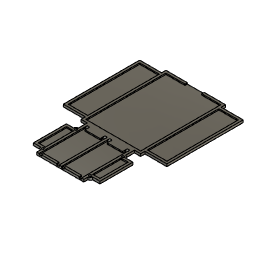
RodogCompartmentsV1 (Autodesk Fusion 360 design; units mm, degrees)
Autodesk Fusion 360 part; units mm, degrees
note: some values were not read from the file. Chosen so that the rebuilt part matches the saved one: which pieces of a blend or face edit are solid. Set by a fixed rule: which sketch regions a step uses.
sketch "Sketch1" plane through (0, 0, 0) normal (0, 0, 1) x (1, 0, 0)
sketch "Sketch2" plane through (0, 0, 0) normal (0, 0, 1) x (1, 0, 0)
  line L0 (25.146, 24.384) -> (-25.146, 24.384)
  line L1 (-25.146, 24.384) -> (-25.146, -24.384)
  line L2 (-25.146, -24.384) -> (25.146, -24.384)
  line L3 (25.146, -24.384) -> (25.146, 24.384)
  line L4 (25.146, 24.384) -> (-25.146, -24.384) construction
  line L5 (-25.146, 24.384) -> (25.146, -24.384) construction
  dimension "d3" = 50.292
  dimension "d4" = 48.768
  constraint horizontal L0
  constraint perpendicular L0 L1
  constraint parallel L0 L2
  constraint parallel L1 L3
  constraint coincident L4 origin
  constraint coincident L5 origin
  measures "d3" distance of L1.end L2.end
  measures "d4" distance of L0.end L1.end
extrude "Extrude1" add sketch "Sketch2" along normal blind 2.54 makes body 1
sketch "Sketch3" plane through (0, 0, 2.54) normal (0, 0, 1) x (-1, 0, 0)
  line L0 (-25.146, 24.384) -> (-25.146, -24.384)
  line L1 (-25.146, -24.384) -> (25.146, -24.384)
  line L2 (25.146, -24.384) -> (25.146, 24.384)
  line L3 (25.146, 24.384) -> (-25.146, 24.384)
  line L4 (-25.146, 24.384) -> (-22.606, 24.384)
  line L5 (-22.606, 24.384) -> (-22.606, 21.844)
  line L6 (-22.606, 21.844) -> (-25.146, 21.844)
  line L7 (-25.146, 21.844) -> (-25.146, 24.384)
  line L8 (-22.606, 21.844) -> (-1.27, 21.844)
  line L9 (-1.27, 21.844) -> (-1.27, -21.844)
  line L10 (-1.27, -21.844) -> (-22.606, -21.844)
  line L11 (-22.606, -21.844) -> (-22.606, 21.844)
  line L12 (-1.27, 21.844) -> (1.27, 21.844)
  line L13 (1.27, 21.844) -> (22.606, 21.844)
  line L14 (22.606, 21.844) -> (22.606, -21.844)
  line L15 (22.606, -21.844) -> (1.27, -21.844)
  line L16 (1.27, -21.844) -> (1.27, 21.844)
  dimension "d7" = 2.54
  dimension "d8" = 2.54
  dimension "d9" = 21.336
  dimension "d10" = 43.688
  dimension "d11" = 2.54
  dimension "d12" = 21.336
  dimension "d13" = 43.688
  constraint horizontal L4
  constraint vertical L5
  constraint horizontal L6
  constraint vertical L7
  constraint coincident L0.start L3.end
  constraint horizontal L8
  constraint vertical L9
  constraint horizontal L10
  constraint vertical L11
  constraint perpendicular L9 L12
  constraint horizontal L13
  constraint vertical L14
  constraint horizontal L15
  constraint vertical L16
  measures "d7" distance of L0.start L4.end
  measures "d8" distance of L0.start L6.end
  measures "d9" distance of L5.end L8.end
  measures "d10" distance of L5.end L10.end
  measures "d11" distance of L8.end L12.end
  measures "d12" distance of L12.end L13.end
  measures "d13" distance of L12.end L15.end
extrude "Extrude2" cut sketch "Sketch3" against normal blind 1.27 contours L8 L9 L10 L11 | L13 L14 L15 L16 bodies 1
sketch "Sketch4" plane through (0, 0, 2.54) normal (0, 0, 1) x (-1, 0, 0)
  line L0 (-1.27, 21.844) -> (-1.27, -21.844)
  line L1 (-1.27, -21.844) -> (-22.606, -21.844)
  line L2 (-22.606, -21.844) -> (-22.606, 21.844)
  line L3 (-22.606, 21.844) -> (-1.27, 21.844)
  line L4 (22.606, 21.844) -> (22.606, -21.844)
  line L5 (22.606, -21.844) -> (1.27, -21.844)
  line L6 (1.27, -21.844) -> (1.27, 21.844)
  line L7 (1.27, 21.844) -> (22.606, 21.844)
  line L8 (-25.146, 24.384) -> (-25.146, -24.384)
  line L9 (-25.146, -24.384) -> (25.146, -24.384)
  line L10 (25.146, -24.384) -> (25.146, 24.384)
  line L11 (25.146, 24.384) -> (-25.146, 24.384)
  line L12 (-22.606, 21.844) -> (-20.066, 21.844)
  line L13 (-20.066, 21.844) -> (-20.066, 24.384)
  line L14 (-20.066, 24.384) -> (-22.606, 24.384)
  line L15 (-22.606, 24.384) -> (-22.606, 21.844)
  line L16 (-1.27, 21.844) -> (-3.81, 21.844)
  line L17 (-3.81, 21.844) -> (-3.81, 24.384)
  line L18 (-3.81, 24.384) -> (-1.27, 24.384)
  line L19 (-1.27, 24.384) -> (-1.27, 21.844)
  line L20 (-22.606, -21.844) -> (-20.066, -21.844)
  line L21 (-20.066, -21.844) -> (-20.066, -24.384)
  line L22 (-20.066, -24.384) -> (-22.606, -24.384)
  line L23 (-22.606, -24.384) -> (-22.606, -21.844)
  line L24 (-1.27, -21.844) -> (-3.81, -21.844)
  line L25 (-3.81, -21.844) -> (-3.81, -24.384)
  line L26 (-3.81, -24.384) -> (-1.27, -24.384)
  line L27 (-1.27, -24.384) -> (-1.27, -21.844)
  dimension "d16" = 2.54
  dimension "d17" = 2.54
  dimension "d18" = 2.54
  dimension "d19" = 2.54
  dimension "d20" = 2.54
  dimension "d21" = 2.54
  constraint horizontal L12
  constraint vertical L13
  constraint horizontal L14
  constraint vertical L15
  constraint coincident L2.end L3.start
  constraint horizontal L16
  constraint vertical L17
  constraint horizontal L18
  constraint vertical L19
  constraint coincident L0.start L3.end
  constraint horizontal L20
  constraint vertical L21
  constraint horizontal L22
  constraint vertical L23
  constraint coincident L1.end L2.start
  constraint horizontal L24
  constraint vertical L25
  constraint horizontal L26
  constraint vertical L27
  constraint coincident L0.end L1.start
  measures "d16" distance of L2.end L12.end
  measures "d17" distance of L0.start L16.end
  measures "d18" distance of L0.start L18.end
  measures "d19" distance of L1.end L20.end
  measures "d20" distance of L1.end L22.end
  measures "d21" distance of L0.end L24.end
extrude "Extrude3" cut sketch "Sketch4" against normal blind 1.27 contours L3 L11 L16 L17 L18 L19 | L1 L9 L24 L25 L26 L27 | L3 L11 L12 L13 L14 L15 | L1 L9 L20 L21 L22 L23 bodies 1
sketch "Sketch5" plane through (0, 0, 2.54) normal (0, 0, 1) x (-1, 0, 0)
  line L0 (-1.27, 24.384) -> (-1.27, -24.384)
  line L1 (-1.27, -24.384) -> (25.146, -24.384)
  line L2 (25.146, -24.384) -> (25.146, 24.384)
  line L3 (25.146, 24.384) -> (-1.27, 24.384)
  line L4 (22.606, 21.844) -> (22.606, -21.844)
  line L5 (22.606, -21.844) -> (1.27, -21.844)
  line L6 (1.27, -21.844) -> (1.27, 21.844)
  line L7 (1.27, 21.844) -> (22.606, 21.844)
  line L8 (1.27, 21.844) -> (3.81, 21.844)
  line L9 (3.81, 21.844) -> (3.81, 24.384)
  line L10 (3.81, 24.384) -> (1.27, 24.384)
  line L11 (1.27, 24.384) -> (1.27, 21.844)
  line L12 (22.606, 21.844) -> (20.066, 21.844)
  line L13 (20.066, 21.844) -> (20.066, 24.384)
  line L14 (20.066, 24.384) -> (22.606, 24.384)
  line L15 (22.606, 24.384) -> (22.606, 21.844)
  line L16 (1.27, -21.844) -> (3.81, -21.844)
  line L17 (3.81, -21.844) -> (3.81, -24.384)
  line L18 (3.81, -24.384) -> (1.27, -24.384)
  line L19 (1.27, -24.384) -> (1.27, -21.844)
  line L20 (22.606, -21.844) -> (20.066, -21.844)
  line L21 (20.066, -21.844) -> (20.066, -24.384)
  line L22 (20.066, -24.384) -> (22.606, -24.384)
  line L23 (22.606, -24.384) -> (22.606, -21.844)
  dimension "d24" = 2.54
  dimension "d25" = 2.54
  dimension "d26" = 2.54
  dimension "d27" = 2.54
  constraint horizontal L8
  constraint vertical L9
  constraint horizontal L10
  constraint vertical L11
  constraint coincident L6.end L7.start
  constraint horizontal L12
  constraint vertical L13
  constraint horizontal L14
  constraint vertical L15
  constraint coincident L4.start L7.end
  constraint horizontal L16
  constraint vertical L17
  constraint horizontal L18
  constraint vertical L19
  constraint coincident L5.end L6.start
  constraint horizontal L20
  constraint vertical L21
  constraint horizontal L22
  constraint vertical L23
  constraint coincident L4.end L5.start
  measures "d24" distance of L6.end L8.end
  measures "d25" distance of L4.start L12.end
  measures "d26" distance of L5.end L16.end
  measures "d27" distance of L4.end L20.end
extrude "Extrude4" cut sketch "Sketch5" against normal blind 1.27 contours L3 L7 L8 L9 L10 L11 | L1 L5 L16 L17 L18 L19 | L3 L7 L12 L13 L14 L15 | L1 L5 L20 L21 L22 L23 bodies 1
sketch "Sketch6" plane through (25.146, 0, 0) normal (1, 0, 0) x (0, 1, 0)
  line L0 (-24.384, 0) -> (24.384, 0)
  line L1 (24.384, 0) -> (24.384, 2.54)
  line L2 (24.384, 2.54) -> (-24.384, 2.54)
  line L3 (-24.384, 2.54) -> (-24.384, 0)
  line L4 (-24.384, 2.54) -> (0, 2.54)
  line L5 (0, 2.54) -> (0, 1.27)
  line L6 (15.0368, 2.54) -> (-15.0368, 2.54)
  line L7 (-15.0368, 2.54) -> (-15.0368, 0)
  line L8 (-15.0368, 0) -> (15.0368, 0)
  line L9 (15.0368, 0) -> (15.0368, 2.54)
  line L10 (15.0368, 2.54) -> (-15.0368, 0) construction
  line L11 (-15.0368, 2.54) -> (15.0368, 0) construction
  point P0 (0, 1.27)
  dimension "d30" = 24.384
  dimension "d31" = 1.27
  dimension "d32" = 30.0736
  dimension "d33" = 2.54
  constraint coincident L2.end L3.start
  constraint perpendicular L3 L4
  constraint perpendicular L4 L5
  constraint horizontal L6
  constraint perpendicular L6 L7
  constraint parallel L6 L8
  constraint parallel L7 L9
  constraint coincident L10 P0
  constraint coincident L11 P0
  constraint coincident P0 L5.end
  measures "d30" distance of L2.end L4.end
  measures "d31" distance of L4.end P0
  measures "d32" distance of L7.end L8.end
  measures "d33" distance of L6.end L7.end
extrude "Extrude5" add sketch "Sketch6" along normal blind 10.287 contours L0 L2 L4 L6 L7 L8 L9 bodies 1
extrude "Extrude6" add 1 faces at (28.575, -15.0368, 1.6933) along direction (0, -1, 0) blind 2.54 on bodies 1 bodies 1
extrude "Extrude7" add 1 faces at (28.575, 15.0368, 0.8467) along direction (0, 1, 0) blind 2.54 on bodies 1 bodies 1
sketch "Sketch7" plane through (0, 0, 2.54) normal (0, 0, 1) x (-1, 0, 0)
  line L0 (-22.606, -24.384) -> (-22.606, 24.384)
  line L1 (-22.606, 24.384) -> (-25.146, 24.384)
  line L2 (-25.146, 24.384) -> (-25.146, 17.5768)
  line L3 (-25.146, 17.5768) -> (-35.433, 17.5768)
  line L4 (-35.433, 17.5768) -> (-35.433, -17.5768)
  line L5 (-35.433, -17.5768) -> (-25.146, -17.5768)
  line L6 (-25.146, -17.5768) -> (-25.146, -24.384)
  line L7 (-25.146, -24.384) -> (-22.606, -24.384)
  line L8 (-35.433, 17.5768) -> (-32.893, 17.5768)
  line L9 (-32.893, 17.5768) -> (-32.893, 15.0368)
  line L10 (-32.893, 15.0368) -> (-35.433, 15.0368)
  line L11 (-35.433, 15.0368) -> (-35.433, 17.5768)
  line L12 (-32.893, 15.0368) -> (-25.146, 15.0368)
  line L13 (-25.146, 15.0368) -> (-25.146, -15.0368)
  line L14 (-25.146, -15.0368) -> (-32.893, -15.0368)
  line L15 (-32.893, -15.0368) -> (-32.893, 15.0368)
  dimension "d40" = 2.54
  dimension "d41" = 2.54
  dimension "d42" = 7.747
  dimension "d43" = 30.0736
  constraint horizontal L8
  constraint vertical L9
  constraint horizontal L10
  constraint vertical L11
  constraint coincident L3.end L4.start
  constraint horizontal L12
  constraint vertical L13
  constraint horizontal L14
  constraint vertical L15
  measures "d40" distance of L3.end L8.end
  measures "d41" distance of L3.end L10.end
  measures "d42" distance of L9.end L12.end
  measures "d43" distance of L9.end L14.end
extrude "Extrude8" cut sketch "Sketch7" against normal blind 1.27 contours L12 L13 L14 L15 bodies 1
sketch "Sketch8" plane through (-25.146, 0, 0) normal (-1, 0, 0) x (0, -1, 0)
  line L0 (-24.384, 0) -> (24.384, 0)
  line L1 (24.384, 0) -> (24.384, 2.54)
  line L2 (24.384, 2.54) -> (-24.384, 2.54)
  line L3 (-24.384, 2.54) -> (-24.384, 0)
  line L4 (-24.384, 2.54) -> (0, 2.54)
  line L5 (0, 2.54) -> (0, 1.27)
  line L6 (-17.5768, 0) -> (17.5768, 0)
  line L7 (17.5768, 0) -> (17.5768, 2.54)
  line L8 (17.5768, 2.54) -> (-17.5768, 2.54)
  line L9 (-17.5768, 2.54) -> (-17.5768, 0)
  line L10 (-17.5768, 0) -> (17.5768, 2.54) construction
  line L11 (17.5768, 0) -> (-17.5768, 2.54) construction
  point P0 (0, 1.27)
  dimension "d46" = 24.384
  dimension "d47" = 1.27
  dimension "d48" = 35.1536
  constraint coincident L2.end L3.start
  constraint perpendicular L3 L4
  constraint perpendicular L4 L5
  constraint horizontal L6
  constraint perpendicular L6 L7
  constraint parallel L6 L8
  constraint parallel L7 L9
  constraint coincident L10 P0
  constraint coincident L11 P0
  constraint coincident P0 L5.end
  measures "d46" distance of L2.end L4.end
  measures "d47" distance of L4.end P0
  measures "d48" distance of L7.end L8.end
extrude "Extrude9" add sketch "Sketch8" along normal blind 10.287 contours L0 L2 L4 L6 L7 L8 L9 bodies 1
sketch "Sketch9" plane through (0, 0, 2.54) normal (0, 0, 1) x (-1, 0, 0)
  line L0 (22.606, 24.384) -> (22.606, -24.384)
  line L1 (22.606, -24.384) -> (25.146, -24.384)
  line L2 (25.146, -24.384) -> (25.146, -17.5768)
  line L3 (25.146, -17.5768) -> (35.433, -17.5768)
  line L4 (35.433, -17.5768) -> (35.433, 17.5768)
  line L5 (35.433, 17.5768) -> (25.146, 17.5768)
  line L6 (25.146, 17.5768) -> (25.146, 24.384)
  line L7 (25.146, 24.384) -> (22.606, 24.384)
  line L8 (35.433, 17.5768) -> (32.893, 17.5768)
  line L9 (32.893, 17.5768) -> (32.893, 15.0368)
  line L10 (32.893, 15.0368) -> (35.433, 15.0368)
  line L11 (35.433, 15.0368) -> (35.433, 17.5768)
  line L12 (32.893, 15.0368) -> (24.003, 15.0368)
  line L13 (24.003, 15.0368) -> (24.003, -15.0368)
  line L14 (24.003, -15.0368) -> (32.893, -15.0368)
  line L15 (32.893, -15.0368) -> (32.893, 15.0368)
  dimension "d51" = 2.54
  dimension "d52" = 2.54
  dimension "d53" = 8.89
  dimension "d54" = 30.0736
  constraint horizontal L8
  constraint vertical L9
  constraint horizontal L10
  constraint vertical L11
  constraint coincident L4.end L5.start
  constraint horizontal L12
  constraint vertical L13
  constraint horizontal L14
  constraint vertical L15
  measures "d51" distance of L4.end L8.end
  measures "d52" distance of L4.end L10.end
  measures "d53" distance of L9.end L12.end
  measures "d54" distance of L9.end L14.end
extrude "Extrude10" cut sketch "Sketch9" against normal blind 1.27 contours L12 L13 L14 L15 bodies 1
extrude "Extrude11" add 1 faces at (-26.9663, -5.0123, 1.27) along direction (0, 0, 1) blind 1.27 on bodies 1 bodies 1
sketch "Sketch11" plane through (0, 0, 2.54) normal (0, 0, 1) x (-1, 0, 0)
  line L0 (22.606, 24.384) -> (22.606, -24.384)
  line L1 (22.606, -24.384) -> (25.146, -24.384)
  line L2 (25.146, -24.384) -> (25.146, -17.5768)
  line L3 (25.146, -17.5768) -> (35.433, -17.5768)
  line L4 (35.433, -17.5768) -> (35.433, 17.5768)
  line L5 (35.433, 17.5768) -> (25.146, 17.5768)
  line L6 (25.146, 17.5768) -> (25.146, 24.384)
  line L7 (25.146, 24.384) -> (22.606, 24.384)
  line L8 (35.433, -17.5768) -> (32.893, -17.5768)
  line L9 (32.893, -17.5768) -> (32.893, -15.0368)
  line L10 (32.893, -15.0368) -> (35.433, -15.0368)
  line L11 (35.433, -15.0368) -> (35.433, -17.5768)
  line L12 (32.893, -15.0368) -> (25.146, -15.0368)
  line L13 (25.146, -15.0368) -> (25.146, 15.0368)
  line L14 (25.146, 15.0368) -> (32.893, 15.0368)
  line L15 (32.893, 15.0368) -> (32.893, -15.0368)
  dimension "d59" = 2.54
  dimension "d60" = 2.54
  dimension "d61" = 7.747
  dimension "d62" = 30.0736
  constraint horizontal L8
  constraint vertical L9
  constraint horizontal L10
  constraint vertical L11
  constraint coincident L3.end L4.start
  constraint horizontal L12
  constraint vertical L13
  constraint horizontal L14
  constraint vertical L15
  measures "d59" distance of L3.end L8.end
  measures "d60" distance of L3.end L10.end
  measures "d61" distance of L9.end L12.end
  measures "d62" distance of L9.end L14.end
extrude "Extrude12" cut sketch "Sketch11" against normal blind 1.27 contours L12 L13 L14 L15 bodies 1
sketch "Sketch13" plane through (0, 17.5768, 0) normal (0, 1, 0) x (-1, 0, 0)
  line L0 (25.146, 2.54) -> (25.146, 0)
  line L1 (25.146, 0) -> (35.433, 0)
  line L2 (35.433, 0) -> (35.433, 2.54)
  line L3 (35.433, 2.54) -> (25.146, 2.54)
  line L4 (25.146, 2.54) -> (27.686, 2.54)
  line L5 (27.686, 2.54) -> (27.686, 0)
  line L6 (27.686, 0) -> (25.146, 0)
  line L7 (25.146, 0) -> (25.146, 2.54)
  dimension "d65" = 2.54
  constraint horizontal L4
  constraint vertical L5
  constraint horizontal L6
  constraint vertical L7
  constraint coincident L0.start L3.end
  measures "d65" distance of L0.start L4.end
extrude "Extrude13" add sketch "Sketch13" along normal blind 2.54 contours L0 L1 L3 L4 L5 L6 L7 bodies 1
sketch "Sketch14" plane through (0, 0, 2.54) normal (0, 0, 1) x (-1, 0, 0)
  circle A0 centre (25.146, -17.5768) radius 1.27
  point P0 (25.146, -17.5768)
  dimension "d68" = 2.54
  constraint coincident P0 A0.centre
  measures "d68" diameter of A0
extrude "Extrude14" cut sketch "Sketch14" against normal blind 1.27 bodies 1
fillet "Fillet1" radius 2.54 1 edges at (-27.686, 20.1168, 1.27) on bodies 1
sketch "Sketch15" plane through (25.146, 0, 0) normal (1, 0, 0) x (0, 1, 0)
  line L0 (17.5768, 2.54) -> (17.5768, 0)
  line L1 (17.5768, 0) -> (24.384, 0)
  line L2 (24.384, 0) -> (24.384, 2.54)
  line L3 (24.384, 2.54) -> (17.5768, 2.54)
  line L4 (17.5768, 2.54) -> (20.1168, 2.54)
  line L5 (20.1168, 2.54) -> (20.1168, 0)
  line L6 (20.1168, 0) -> (17.5768, 0)
  line L7 (17.5768, 0) -> (17.5768, 2.54)
  dimension "d73" = 2.54
  constraint horizontal L4
  constraint vertical L5
  constraint horizontal L6
  constraint vertical L7
  constraint coincident L0.start L3.end
  measures "d73" distance of L0.start L4.end
extrude "Extrude15" add sketch "Sketch15" along normal blind 2.54 contours L0 L1 L3 L4 L5 L6 L7 bodies 1
sketch "Sketch16" plane through (25.146, 0, 0) normal (1, 0, 0) x (0, 1, 0)
  line L0 (-17.5768, 0) -> (-17.5768, 2.54)
  line L1 (-17.5768, 2.54) -> (-24.384, 2.54)
  line L2 (-24.384, 2.54) -> (-24.384, 0)
  line L3 (-24.384, 0) -> (-17.5768, 0)
  line L4 (-17.5768, 2.54) -> (-20.1168, 2.54)
  line L5 (-20.1168, 2.54) -> (-20.1168, 0)
  line L6 (-20.1168, 0) -> (-17.5768, 0)
  line L7 (-17.5768, 0) -> (-17.5768, 2.54)
  dimension "d76" = 2.54
  constraint horizontal L4
  constraint vertical L5
  constraint horizontal L6
  constraint vertical L7
  constraint coincident L0.end L1.start
  measures "d76" distance of L0.end L4.end
extrude "Extrude16" add sketch "Sketch16" along normal blind 2.54 contours L0 L1 L3 L4 L5 L6 L7 bodies 1
sketch "Sketch17" plane through (-25.146, 0, 0) normal (-1, 0, 0) x (0, -1, 0)
  line L0 (17.5768, 2.54) -> (17.5768, 0)
  line L1 (17.5768, 0) -> (24.384, 0)
  line L2 (24.384, 0) -> (24.384, 2.54)
  line L3 (24.384, 2.54) -> (17.5768, 2.54)
  line L4 (17.5768, 2.54) -> (20.1168, 2.54)
  line L5 (20.1168, 2.54) -> (20.1168, 0)
  line L6 (20.1168, 0) -> (17.5768, 0)
  line L7 (17.5768, 0) -> (17.5768, 2.54)
  dimension "d79" = 2.54
  constraint horizontal L4
  constraint vertical L5
  constraint horizontal L6
  constraint vertical L7
  constraint coincident L0.start L3.end
  measures "d79" distance of L0.start L4.end
extrude "Extrude17" add sketch "Sketch17" along normal blind 2.54 contours L0 L1 L3 L4 L5 L6 L7 bodies 1
sketch "Sketch18" plane through (0, 0, 2.54) normal (0, 0, 1) x (-1, 0, 0)
  line L0 (35.433, 17.5768) -> (25.146, 17.5768)
  line L1 (22.606, 24.384) -> (22.606, -24.384)
  line L2 (27.7188, 17.5768) -> (22.606, 17.5768)
  circle A0 centre (25.146, 17.5768) radius 1.27
  line L3 (-27.686, 17.526) -> (-22.606, 17.526)
  circle A1 centre (-25.146, 17.526) radius 1.27
  line L4 (-27.686, -17.526) -> (-22.606, -17.526)
  circle A2 centre (-25.146, -17.526) radius 1.27
  dimension "d82" = 2.54
  dimension "d83" = 2.54
  dimension "d84" = 2.54
  constraint coincident L0 L2.start
  constraint coincident L1 L2.end
  constraint perpendicular L1 L2
  constraint coincident L0.end A0.centre
  constraint horizontal L3
  constraint midpoint L3 A1.centre
  constraint horizontal L4
  constraint midpoint L4 A2.centre
  measures "d82" diameter of A0
  measures "d83" diameter of A1
  measures "d84" diameter of A2
extrude "Extrude18" cut sketch "Sketch18" against normal blind 1.27 bodies 1
fillet "Fillet2" radius 2.54 3 edges at (-27.686, -20.1168, 1.27) (27.686, -20.1168, 1.27) (27.686, 20.1168, 1.27) on bodies 1
sketch "Sketch20" plane through (0, 0, 0) normal (0, 0, 1) x (1, 0, 0)
  circle A0 centre (63.5, 12.7) radius 1.27
  dimension "d89" = 2.54
  measures "d89" diameter of A0
extrude "Extrude19" add sketch "Sketch20" along normal blind 18.034 separate body makes body 2
move_face "MoveFace1" to x (1, 0, 0) y (0, 1, 0) z (0, 0, 1) at (-25.4, 0, 0) 1 faces at (64.0223, 13.8576, 12.0227) on bodies 2
sketch "Sketch23" plane through (0, 0, 0) normal (0, 0, 1) x (1, 0, 0)
  circle A0 centre (38.1, 8.89) radius 1.27
  dimension "d92" = 2.54
  measures "d92" diameter of A0
extrude "Extrude20" add sketch "Sketch23" along normal blind 18.034 separate body makes body 3
copy_body "CopyPasteBodies1" bodies 2 makes body 4
move_body "Move1" bodies 4 to x (1, 0, 0) y (0, 1, 0) z (0, 0, 1) at (0, -7.62, 0)
copy_body "CopyPasteBodies2" bodies 4 makes body 5
move_body "Move2" bodies 5 to x (1, 0, 0) y (0, 1, 0) z (0, 0, 1) at (0, -3.81, 0)
sketch "Sketch24" plane through (0, 24.384, 0) normal (0, 1, 0) x (-1, 0, 0)
  line L0 (22.606, 2.54) -> (22.606, 1.27)
  line L1 (22.606, 1.27) -> (20.066, 1.27)
  line L2 (20.066, 1.27) -> (20.066, 2.54)
  line L3 (20.066, 2.54) -> (3.81, 2.54)
  line L4 (3.81, 2.54) -> (3.81, 1.27)
  line L5 (3.81, 1.27) -> (1.27, 1.27)
  line L6 (1.27, 1.27) -> (1.27, 2.54)
  line L7 (1.27, 2.54) -> (-1.27, 2.54)
  line L8 (-1.27, 2.54) -> (-1.27, 1.27)
  line L9 (-1.27, 1.27) -> (-3.81, 1.27)
  line L10 (-3.81, 1.27) -> (-3.81, 2.54)
  line L11 (-3.81, 2.54) -> (-20.066, 2.54)
  line L12 (-20.066, 2.54) -> (-20.066, 1.27)
  line L13 (-20.066, 1.27) -> (-22.606, 1.27)
  line L14 (-22.606, 1.27) -> (-22.606, 2.54)
  line L15 (-22.606, 2.54) -> (-25.146, 2.54)
  line L16 (-25.146, 2.54) -> (-25.146, 0)
  line L17 (-25.146, 0) -> (25.146, 0)
  line L18 (25.146, 0) -> (25.146, 2.54)
  line L19 (25.146, 2.54) -> (22.606, 2.54)
extrude "Extrude21" add sketch "Sketch24" along normal blind 2.54 bodies 1
sketch "Sketch25" plane through (0, 0, 1.27) normal (0, 0, 1) x (-1, 0, 0)
  line L0 (-1.27, -26.924) -> (-1.27, 24.384)
  line L1 (-1.27, 24.384) -> (-3.81, 24.384)
  line L2 (-3.81, 24.384) -> (-3.81, 21.844)
  line L3 (-3.81, 21.844) -> (-20.066, 21.844)
  line L4 (-20.066, 21.844) -> (-20.066, 24.384)
  line L5 (-20.066, 24.384) -> (-22.606, 24.384)
  line L6 (-22.606, 24.384) -> (-22.606, -26.924)
  line L7 (-22.606, -26.924) -> (-20.066, -26.924)
  line L8 (-20.066, -26.924) -> (-20.066, -21.844)
  line L9 (-20.066, -21.844) -> (-3.81, -21.844)
  line L10 (-3.81, -21.844) -> (-3.81, -26.924)
  line L11 (-3.81, -26.924) -> (-1.27, -26.924)
  line L12 (-22.606, -26.924) -> (-20.066, -26.924)
  line L13 (-20.066, -26.924) -> (-20.066, -24.384)
  line L14 (-20.066, -24.384) -> (-22.606, -24.384)
  line L15 (-22.606, -24.384) -> (-22.606, -26.924)
  line L16 (-1.27, -26.924) -> (-3.81, -26.924)
  line L17 (-3.81, -26.924) -> (-3.81, -24.384)
  line L18 (-3.81, -24.384) -> (-1.27, -24.384)
  line L19 (-1.27, -24.384) -> (-1.27, -26.924)
  dimension "d97" = 2.54
  dimension "d98" = 2.54
  constraint horizontal L12
  constraint vertical L13
  constraint horizontal L14
  constraint vertical L15
  constraint coincident L6.end L7.start
  constraint horizontal L16
  constraint vertical L17
  constraint horizontal L18
  constraint vertical L19
  constraint coincident L0.start L11.end
  measures "d97" distance of L6.end L14.end
  measures "d98" distance of L0.start L18.end
extrude "Extrude22" add sketch "Sketch25" along normal blind 1.27 contours L6 L7 L8 L12 L13 L14 L15 bodies 1
fillet "Fillet3" radius 3.81 1 edges at (21.336, 24.384, 2.54) on bodies 1
sketch "Sketch27" plane through (1.27, 0, 0) normal (1, 0, 0) x (0, 1, 0)
  line L0 (26.924, 2.54) -> (-24.384, 2.54)
  line L1 (-24.384, 2.54) -> (-24.384, 1.27)
  line L2 (-24.384, 1.27) -> (26.924, 1.27)
  line L3 (26.924, 1.27) -> (26.924, 2.54)
  line L4 (26.924, 2.54) -> (24.384, 2.54)
  line L5 (24.384, 2.54) -> (24.384, 1.27)
  line L6 (24.384, 1.27) -> (26.924, 1.27)
  line L7 (26.924, 1.27) -> (26.924, 2.54)
  dimension "d103" = 2.54
  constraint horizontal L4
  constraint vertical L5
  constraint horizontal L6
  constraint vertical L7
  constraint coincident L0.start L3.end
  measures "d103" distance of L0.start L4.end
extrude "Extrude23" add sketch "Sketch27" along normal blind 2.54 contours L0 L2 L3 L4 L5 L6 L7 bodies 1
fillet "Fillet4" radius 3.81 1 edges at (2.54, 24.384, 2.54) on bodies 1
sketch "Sketch28" plane through (-3.81, 0, 0) normal (1, 0, 0) x (0, 1, 0)
  line L0 (26.924, 2.54) -> (21.844, 2.54)
  line L1 (21.844, 2.54) -> (21.844, 1.27)
  line L2 (21.844, 1.27) -> (26.924, 1.27)
  line L3 (26.924, 1.27) -> (26.924, 2.54)
  line L4 (26.924, 2.54) -> (24.384, 2.54)
  line L5 (24.384, 2.54) -> (24.384, 1.27)
  line L6 (24.384, 1.27) -> (26.924, 1.27)
  line L7 (26.924, 1.27) -> (26.924, 2.54)
  dimension "d108" = 2.54
  constraint horizontal L4
  constraint vertical L5
  constraint horizontal L6
  constraint vertical L7
  constraint coincident L0.start L3.end
  measures "d108" distance of L0.start L4.end
extrude "Extrude24" add sketch "Sketch28" along normal blind 2.54 contours L0 L2 L3 L4 L5 L6 L7 bodies 1
fillet "Fillet5" radius 3.81 1 edges at (-2.54, 24.384, 2.54) on bodies 1
sketch "Sketch29" plane through (-22.606, 0, 0) normal (1, 0, 0) x (0, 1, 0)
  line L0 (26.924, 2.54) -> (-24.384, 2.54)
  line L1 (-24.384, 2.54) -> (-24.384, 1.27)
  line L2 (-24.384, 1.27) -> (26.924, 1.27)
  line L3 (26.924, 1.27) -> (26.924, 2.54)
  line L4 (26.924, 2.54) -> (24.384, 2.54)
  line L5 (24.384, 2.54) -> (24.384, 1.27)
  line L6 (24.384, 1.27) -> (26.924, 1.27)
  line L7 (26.924, 1.27) -> (26.924, 2.54)
  dimension "d113" = 2.54
  constraint horizontal L4
  constraint vertical L5
  constraint horizontal L6
  constraint vertical L7
  constraint coincident L0.start L3.end
  measures "d113" distance of L0.start L4.end
extrude "Extrude25" add sketch "Sketch29" along normal blind 2.54 contours L0 L2 L3 L4 L5 L6 L7 bodies 1
sketch "Sketch30" plane through (0, 0, 2.54) normal (0, 0, 1) x (-1, 0, 0)
  line L0 (25.146, -15.0368) -> (25.146, 15.0368)
  line L1 (25.146, 15.0368) -> (32.893, 15.0368)
  line L2 (32.893, 15.0368) -> (32.893, -15.0368)
  line L3 (32.893, -15.0368) -> (25.146, -15.0368)
  circle A0 centre (25.146, -17.5768) radius 1.27
  circle A1 centre (25.146, 17.5768) radius 1.27
  line L4 (3.81, -21.844) -> (3.81, -26.924)
  line L5 (3.81, -26.924) -> (25.146, -26.924)
  line L6 (25.146, -26.924) -> (25.146, -20.1168)
  arc A2 (25.146, -20.1168) -> (27.686, -17.5768) centre (25.146, -17.5768) ccw
  line L7 (27.686, -17.5768) -> (35.433, -17.5768)
  line L8 (35.433, -17.5768) -> (35.433, 17.5768)
  line L9 (35.433, 17.5768) -> (27.686, 17.5768)
  arc A3 (27.686, 17.5768) -> (25.146, 20.1168) centre (25.146, 17.5768) ccw
  line L10 (25.146, 20.1168) -> (25.146, 24.384)
  line L11 (25.146, 24.384) -> (22.606, 24.384)
  line L12 (22.606, 24.384) -> (22.606, -24.384)
  line L13 (22.606, -24.384) -> (20.066, -24.384)
  line L14 (20.066, -24.384) -> (20.066, -21.844)
  line L15 (20.066, -21.844) -> (3.81, -21.844)
fillet "Fillet6" radius 3.81 1 edges at (-21.336, 24.384, 2.54) on bodies 1
extrude "Extrude26" add 1 faces at (-1.27, 26.924, 0.8467) along direction (0, 1, 0) blind 1.27 on bodies 1 bodies 1
sketch "Sketch31" plane through (0, 28.194, 0) normal (0, 1, 0) x (-1, 0, 0)
  line L0 (25.146, 2.54) -> (-25.146, 2.54)
  line L1 (-25.146, 2.54) -> (-25.146, 0)
  line L2 (-25.146, 0) -> (25.146, 0)
  line L3 (25.146, 0) -> (25.146, 2.54)
extrude "Extrude27" add sketch "Sketch31" along normal blind 1.27 bodies 1
sketch "Sketch32" plane through (0, 0, 0) normal (0, 0, 1) x (1, 0, 0)
  line L0 (0, 29.464) -> (29.2354, 29.464)
  line L1 (0, 29.464) -> (-29.2354, 29.464)
  line L2 (29.2354, 29.464) -> (31.7754, 29.464)
  line L3 (-29.2354, 29.464) -> (-31.7754, 29.464)
  line L4 (31.7754, 29.464) -> (-31.7754, 29.464)
  line L5 (-31.7754, 29.464) -> (-31.7754, 119.9388)
  line L6 (-31.7754, 119.9388) -> (31.7754, 119.9388)
  line L7 (31.7754, 119.9388) -> (31.7754, 29.464)
  dimension "d123" = 29.2354
  dimension "d124" = 29.2354
  dimension "d125" = 2.54
  dimension "d126" = 2.54
  dimension "d127" = 63.5508
  dimension "d128" = 90.4748
  constraint parallel L0 L2
  constraint parallel L1 L3
  constraint horizontal L4
  constraint vertical L5
  constraint horizontal L6
  constraint vertical L7
  measures "d123" distance of L0.start L0.end
  measures "d124" distance of L0.start L1.end
  measures "d125" distance of L0.end L2.end
  measures "d126" distance of L1.end L3.end
  measures "d127" distance of L2.end L3.end
  measures "d128" distance of L2.end L6.end
extrude "Extrude28" add sketch "Sketch32" along normal blind 2.54 bodies 1
sketch "Sketch33" plane through (0, 0, 2.54) normal (0, 0, 1) x (-1, 0, 0)
  circle A0 centre (-25.146, -17.526) radius 1.27
  circle A1 centre (-25.146, 17.526) radius 1.27
  line L0 (-25.146, 15.0368) -> (-25.146, -15.0368)
  line L1 (-25.146, -15.0368) -> (-32.893, -15.0368)
  line L2 (-32.893, -15.0368) -> (-32.893, 15.0368)
  line L3 (-32.893, 15.0368) -> (-25.146, 15.0368)
  circle A2 centre (25.146, 17.5768) radius 1.27
  circle A3 centre (25.146, -17.5768) radius 1.27
  line L4 (25.146, -15.0368) -> (25.146, 15.0368)
  line L5 (25.146, 15.0368) -> (32.893, 15.0368)
  line L6 (32.893, 15.0368) -> (32.893, -15.0368)
  line L7 (32.893, -15.0368) -> (25.146, -15.0368)
  line L8 (22.606, 24.384) -> (22.606, -26.924)
  line L9 (22.606, -26.924) -> (20.066, -26.924)
  line L10 (20.066, -26.924) -> (20.066, -21.844)
  line L11 (20.066, -21.844) -> (3.81, -21.844)
  line L12 (3.81, -21.844) -> (3.81, -26.924)
  line L13 (3.81, -26.924) -> (1.27, -26.924)
  line L14 (1.27, -26.924) -> (1.27, 24.384)
  line L15 (1.27, 24.384) -> (-1.27, 24.384)
  line L16 (-1.27, 24.384) -> (-1.27, -26.924)
  line L17 (-1.27, -26.924) -> (-3.81, -26.924)
  line L18 (-3.81, -26.924) -> (-3.81, -21.844)
  line L19 (-3.81, -21.844) -> (-20.066, -21.844)
  line L20 (-20.066, -21.844) -> (-20.066, -26.924)
  line L21 (-20.066, -26.924) -> (-22.606, -26.924)
  line L22 (-22.606, -26.924) -> (-22.606, 24.384)
  line L23 (-22.606, 24.384) -> (-25.146, 24.384)
  line L24 (-25.146, 24.384) -> (-25.146, 20.1168)
  arc A4 (-25.146, 20.1168) -> (-27.686, 17.5768) centre (-25.146, 17.5768) ccw
  line L25 (-27.686, 17.5768) -> (-35.433, 17.5768)
  line L26 (-35.433, 17.5768) -> (-35.433, -17.5768)
  line L27 (-35.433, -17.5768) -> (-27.686, -17.5768)
  arc A5 (-27.686, -17.5768) -> (-25.146, -20.1168) centre (-25.146, -17.5768) ccw
  line L28 (-25.146, -20.1168) -> (-25.146, -29.464)
  line L29 (-25.146, -29.464) -> (-31.7754, -29.464)
  line L30 (-31.7754, -29.464) -> (-31.7754, -119.9388)
  line L31 (-31.7754, -119.9388) -> (31.7754, -119.9388)
  line L32 (31.7754, -119.9388) -> (31.7754, -29.464)
  line L33 (31.7754, -29.464) -> (25.146, -29.464)
  line L34 (25.146, -29.464) -> (25.146, -20.1168)
  arc A6 (25.146, -20.1168) -> (27.686, -17.5768) centre (25.146, -17.5768) ccw
  line L35 (27.686, -17.5768) -> (35.433, -17.5768)
  line L36 (35.433, -17.5768) -> (35.433, 17.5768)
  line L37 (35.433, 17.5768) -> (27.686, 17.5768)
  arc A7 (27.686, 17.5768) -> (25.146, 20.1168) centre (25.146, 17.5768) ccw
  line L38 (25.146, 20.1168) -> (25.146, 24.384)
  line L39 (25.146, 24.384) -> (22.606, 24.384)
  line L40 (-31.7754, -119.9388) -> (-29.2354, -119.9388)
  line L41 (-29.2354, -119.9388) -> (-29.2354, -117.3988)
  line L42 (-29.2354, -117.3988) -> (-31.7754, -117.3988)
  line L43 (-31.7754, -117.3988) -> (-31.7754, -119.9388)
  line L44 (31.7754, -29.464) -> (29.2354, -29.464)
  line L45 (29.2354, -29.464) -> (29.2354, -32.004)
  line L46 (29.2354, -32.004) -> (31.7754, -32.004)
  line L47 (31.7754, -32.004) -> (31.7754, -29.464)
  line L48 (29.2354, -32.004) -> (-29.2354, -32.004)
  line L49 (-29.2354, -32.004) -> (-29.2354, -117.3988)
  line L50 (-29.2354, -117.3988) -> (29.2354, -117.3988)
  line L51 (29.2354, -117.3988) -> (29.2354, -32.004)
  dimension "d131" = 2.54
  dimension "d132" = 2.54
  dimension "d133" = 2.54
  dimension "d134" = 2.54
  constraint horizontal L40
  constraint vertical L41
  constraint horizontal L42
  constraint vertical L43
  constraint coincident L30.end L31.start
  constraint horizontal L44
  constraint vertical L45
  constraint horizontal L46
  constraint vertical L47
  constraint coincident L32.end L33.start
  constraint horizontal L48
  constraint vertical L49
  constraint horizontal L50
  constraint vertical L51
  measures "d131" distance of L30.end L40.end
  measures "d132" distance of L30.end L42.end
  measures "d133" distance of L32.end L44.end
  measures "d134" distance of L32.end L46.end
extrude "Extrude29" cut sketch "Sketch33" against normal blind 1.27 contours L48 L49 L50 L51 bodies 1
sketch "Sketch34" plane through (0, 119.9388, 0) normal (0, 1, 0) x (-1, 0, 0)
  line L0 (-31.7754, 0) -> (31.7754, 0)
  line L1 (31.7754, 0) -> (31.7754, 2.54)
  line L2 (31.7754, 2.54) -> (-31.7754, 2.54)
  line L3 (-31.7754, 2.54) -> (-31.7754, 0)
  line L4 (29.2354, 2.54, -2.54) -> (-29.2354, 2.54, -2.54)
  line L5 (0, 2.54, -2.54) -> (-8.89, 2.54, -2.54)
  line L6 (0, 2.54, -2.54) -> (8.89, 2.54, -2.54)
  dimension "d137" = 8.89
  dimension "d138" = 8.89
sketch "Sketch35" plane through (0, 0, 2.54) normal (0, 0, 1) x (-1, 0, 0)
  line L0 (-29.2354, -32.004) -> (29.2354, -32.004)
  line L1 (29.2354, -32.004) -> (29.2354, -117.3988)
  line L2 (29.2354, -117.3988) -> (-29.2354, -117.3988)
  line L3 (-29.2354, -117.3988) -> (-29.2354, -32.004)
  circle A0 centre (-25.146, -17.526) radius 1.27
  circle A1 centre (-25.146, 17.526) radius 1.27
  line L4 (-25.146, 15.0368) -> (-25.146, -15.0368)
  line L5 (-25.146, -15.0368) -> (-32.893, -15.0368)
  line L6 (-32.893, -15.0368) -> (-32.893, 15.0368)
  line L7 (-32.893, 15.0368) -> (-25.146, 15.0368)
  circle A2 centre (25.146, 17.5768) radius 1.27
  circle A3 centre (25.146, -17.5768) radius 1.27
  line L8 (25.146, -15.0368) -> (25.146, 15.0368)
  line L9 (25.146, 15.0368) -> (32.893, 15.0368)
  line L10 (32.893, 15.0368) -> (32.893, -15.0368)
  line L11 (32.893, -15.0368) -> (25.146, -15.0368)
  line L12 (22.606, 24.384) -> (22.606, -26.924)
  line L13 (22.606, -26.924) -> (20.066, -26.924)
  line L14 (20.066, -26.924) -> (20.066, -21.844)
  line L15 (20.066, -21.844) -> (3.81, -21.844)
  line L16 (3.81, -21.844) -> (3.81, -26.924)
  line L17 (3.81, -26.924) -> (1.27, -26.924)
  line L18 (1.27, -26.924) -> (1.27, 24.384)
  line L19 (1.27, 24.384) -> (-1.27, 24.384)
  line L20 (-1.27, 24.384) -> (-1.27, -26.924)
  line L21 (-1.27, -26.924) -> (-3.81, -26.924)
  line L22 (-3.81, -26.924) -> (-3.81, -21.844)
  line L23 (-3.81, -21.844) -> (-20.066, -21.844)
  line L24 (-20.066, -21.844) -> (-20.066, -26.924)
  line L25 (-20.066, -26.924) -> (-22.606, -26.924)
  line L26 (-22.606, -26.924) -> (-22.606, 24.384)
  line L27 (-22.606, 24.384) -> (-25.146, 24.384)
  line L28 (-25.146, 24.384) -> (-25.146, 20.1168)
  arc A4 (-25.146, 20.1168) -> (-27.686, 17.5768) centre (-25.146, 17.5768) ccw
  line L29 (-27.686, 17.5768) -> (-35.433, 17.5768)
  line L30 (-35.433, 17.5768) -> (-35.433, -17.5768)
  line L31 (-35.433, -17.5768) -> (-27.686, -17.5768)
  arc A5 (-27.686, -17.5768) -> (-25.146, -20.1168) centre (-25.146, -17.5768) ccw
  line L32 (-25.146, -20.1168) -> (-25.146, -29.464)
  line L33 (-25.146, -29.464) -> (-31.7754, -29.464)
  line L34 (-31.7754, -29.464) -> (-31.7754, -119.9388)
  line L35 (-31.7754, -119.9388) -> (31.7754, -119.9388)
  line L36 (31.7754, -119.9388) -> (31.7754, -29.464)
  line L37 (31.7754, -29.464) -> (25.146, -29.464)
  line L38 (25.146, -29.464) -> (25.146, -20.1168)
  arc A6 (25.146, -20.1168) -> (27.686, -17.5768) centre (25.146, -17.5768) ccw
  line L39 (27.686, -17.5768) -> (35.433, -17.5768)
  line L40 (35.433, -17.5768) -> (35.433, 17.5768)
  line L41 (35.433, 17.5768) -> (27.686, 17.5768)
  arc A7 (27.686, 17.5768) -> (25.146, 20.1168) centre (25.146, 17.5768) ccw
  line L42 (25.146, 20.1168) -> (25.146, 24.384)
  line L43 (25.146, 24.384) -> (22.606, 24.384)
  line L44 (-8.89, -117.3988) -> (8.89, -117.3988)
  line L45 (8.89, -117.3988) -> (8.89, -119.9388)
  line L46 (8.89, -119.9388) -> (-8.89, -119.9388)
  line L47 (-8.89, -119.9388) -> (-8.89, -117.3988)
  point P0 (-8.89, -117.3988)
  dimension "d139" = 17.78
  constraint horizontal L44
  constraint vertical L45
  constraint horizontal L46
  constraint vertical L47
  constraint coincident P0 L44.start
  measures "d139" distance of P0 L44.end
extrude "Extrude30" cut sketch "Sketch35" against normal blind 1.27 contours L2 L35 L44 L45 L46 L47 bodies 1
sketch "Sketch36" plane through (31.7754, 0, 0) normal (1, 0, 0) x (0, 1, 0)
  line L0 (29.464, 0) -> (119.9388, 0)
  line L1 (119.9388, 0) -> (119.9388, 2.54)
  line L2 (119.9388, 2.54) -> (29.464, 2.54)
  line L3 (29.464, 2.54) -> (29.464, 0)
  line L4 (29.464, 0) -> (74.7014, 0)
  line L5 (74.7014, 0) -> (74.7014, 1.27)
  line L6 (36.6014, 2.54) -> (112.8014, 2.54)
  line L7 (112.8014, 2.54) -> (112.8014, 0)
  line L8 (112.8014, 0) -> (36.6014, 0)
  line L9 (36.6014, 0) -> (36.6014, 2.54)
  line L10 (36.6014, 2.54) -> (112.8014, 0) construction
  line L11 (112.8014, 2.54) -> (36.6014, 0) construction
  point P0 (74.7014, 1.27)
  dimension "d142" = 45.2374
  dimension "d143" = 1.27
  dimension "d144" = 76.2
  dimension "d145" = 2.54
  constraint coincident L0.start L3.end
  constraint perpendicular L1 L4
  constraint perpendicular L4 L5
  constraint horizontal L6
  constraint perpendicular L6 L7
  constraint parallel L6 L8
  constraint parallel L7 L9
  constraint coincident L10 P0
  constraint coincident L11 P0
  constraint coincident P0 L5.end
  measures "d142" distance of L0.start L4.end
  measures "d143" distance of L4.end P0
  measures "d144" distance of L7.end L8.end
  measures "d145" distance of L6.end L7.end
extrude "Extrude31" add sketch "Sketch36" along normal blind 23.368 contours L0 L2 L4 L6 L7 L8 L9 bodies 1
extrude "Extrude32" add 1 faces at (39.5647, 112.8014, 1.6933) along direction (0, 1, 0) blind 2.54 on bodies 1 bodies 1
extrude "Extrude33" add 1 faces at (39.5647, 36.6014, 0.8467) along direction (0, -1, 0) blind 2.54 on bodies 1 bodies 1
sketch "Sketch37" plane through (-31.7754, 0, 0) normal (-1, 0, 0) x (0, -1, 0)
  line L0 (-119.9388, 0) -> (-29.464, 0)
  line L1 (-29.464, 0) -> (-29.464, 2.54)
  line L2 (-29.464, 2.54) -> (-119.9388, 2.54)
  line L3 (-119.9388, 2.54) -> (-119.9388, 0)
  line L4 (-119.9388, 0) -> (-74.7014, 0)
  line L5 (-74.7014, 0) -> (-74.7014, 1.27)
  line L6 (-115.3414, 2.54) -> (-34.0614, 2.54)
  line L7 (-34.0614, 2.54) -> (-34.0614, 0)
  line L8 (-34.0614, 0) -> (-115.3414, 0)
  line L9 (-115.3414, 0) -> (-115.3414, 2.54)
  line L10 (-115.3414, 2.54) -> (-34.0614, 0) construction
  line L11 (-34.0614, 2.54) -> (-115.3414, 0) construction
  point P0 (-74.7014, 1.27)
  dimension "d152" = 45.2374
  dimension "d153" = 1.27
  dimension "d154" = 81.28
  constraint coincident L0.start L3.end
  constraint perpendicular L1 L4
  constraint perpendicular L2 L5
  constraint horizontal L6
  constraint perpendicular L6 L7
  constraint parallel L6 L8
  constraint parallel L7 L9
  constraint coincident L10 P0
  constraint coincident L11 P0
  constraint coincident P0 L5.end
  measures "d152" distance of L0.start L4.end
  measures "d153" distance of L4.end P0
  measures "d154" distance of L7.end L8.end
extrude "Extrude34" add sketch "Sketch37" along normal blind 23.368 contours L0 L2 L4 L6 L7 L8 L9 bodies 1
sketch "Sketch38" plane through (0, 0, 2.54) normal (0, 0, 1) x (-1, 0, 0)
  line L0 (8.89, -117.3988) -> (8.89, -119.9388)
  line L1 (8.89, -119.9388) -> (31.7754, -119.9388)
  line L2 (31.7754, -119.9388) -> (31.7754, -115.3414)
  line L3 (31.7754, -115.3414) -> (55.1434, -115.3414)
  line L4 (55.1434, -115.3414) -> (55.1434, -34.0614)
  line L5 (55.1434, -34.0614) -> (31.7754, -34.0614)
  line L6 (31.7754, -34.0614) -> (31.7754, -29.464)
  line L7 (31.7754, -29.464) -> (25.146, -29.464)
  line L8 (25.146, -29.464) -> (25.146, -20.1168)
  arc A0 (25.146, -20.1168) -> (27.686, -17.5768) centre (25.146, -17.5768) ccw
  line L9 (27.686, -17.5768) -> (35.433, -17.5768)
  line L10 (35.433, -17.5768) -> (35.433, 17.5768)
  line L11 (35.433, 17.5768) -> (27.686, 17.5768)
  arc A1 (27.686, 17.5768) -> (25.146, 20.1168) centre (25.146, 17.5768) ccw
  line L12 (25.146, 20.1168) -> (25.146, 24.384)
  line L13 (25.146, 24.384) -> (22.606, 24.384)
  line L14 (22.606, 24.384) -> (22.606, -26.924)
  line L15 (22.606, -26.924) -> (20.066, -26.924)
  line L16 (20.066, -26.924) -> (20.066, -21.844)
  line L17 (20.066, -21.844) -> (3.81, -21.844)
  line L18 (3.81, -21.844) -> (3.81, -26.924)
  line L19 (3.81, -26.924) -> (1.27, -26.924)
  line L20 (1.27, -26.924) -> (1.27, 24.384)
  line L21 (1.27, 24.384) -> (-1.27, 24.384)
  line L22 (-1.27, 24.384) -> (-1.27, -26.924)
  line L23 (-1.27, -26.924) -> (-3.81, -26.924)
  line L24 (-3.81, -26.924) -> (-3.81, -21.844)
  line L25 (-3.81, -21.844) -> (-20.066, -21.844)
  line L26 (-20.066, -21.844) -> (-20.066, -26.924)
  line L27 (-20.066, -26.924) -> (-22.606, -26.924)
  line L28 (-22.606, -26.924) -> (-22.606, 24.384)
  line L29 (-22.606, 24.384) -> (-25.146, 24.384)
  line L30 (-25.146, 24.384) -> (-25.146, 20.1168)
  arc A2 (-25.146, 20.1168) -> (-27.686, 17.5768) centre (-25.146, 17.5768) ccw
  line L31 (-27.686, 17.5768) -> (-35.433, 17.5768)
  line L32 (-35.433, 17.5768) -> (-35.433, -17.5768)
  line L33 (-35.433, -17.5768) -> (-27.686, -17.5768)
  arc A3 (-27.686, -17.5768) -> (-25.146, -20.1168) centre (-25.146, -17.5768) ccw
  line L34 (-25.146, -20.1168) -> (-25.146, -29.464)
  line L35 (-25.146, -29.464) -> (-31.7754, -29.464)
  line L36 (-31.7754, -29.464) -> (-31.7754, -34.0614)
  line L37 (-31.7754, -34.0614) -> (-55.1434, -34.0614)
  line L38 (-55.1434, -34.0614) -> (-55.1434, -115.3414)
  line L39 (-55.1434, -115.3414) -> (-31.7754, -115.3414)
  line L40 (-31.7754, -115.3414) -> (-31.7754, -119.9388)
  line L41 (-31.7754, -119.9388) -> (-8.89, -119.9388)
  line L42 (-8.89, -119.9388) -> (-8.89, -117.3988)
  line L43 (-8.89, -117.3988) -> (-29.2354, -117.3988)
  line L44 (-29.2354, -117.3988) -> (-29.2354, -32.004)
  line L45 (-29.2354, -32.004) -> (29.2354, -32.004)
  line L46 (29.2354, -32.004) -> (29.2354, -117.3988)
  line L47 (29.2354, -117.3988) -> (8.89, -117.3988)
  line L48 (25.146, -15.0368) -> (25.146, 15.0368)
  line L49 (25.146, 15.0368) -> (32.893, 15.0368)
  line L50 (32.893, 15.0368) -> (32.893, -15.0368)
  line L51 (32.893, -15.0368) -> (25.146, -15.0368)
  circle A4 centre (25.146, -17.5768) radius 1.27
  circle A5 centre (25.146, 17.5768) radius 1.27
  line L52 (-25.146, 15.0368) -> (-25.146, -15.0368)
  line L53 (-25.146, -15.0368) -> (-32.893, -15.0368)
  line L54 (-32.893, -15.0368) -> (-32.893, 15.0368)
  line L55 (-32.893, 15.0368) -> (-25.146, 15.0368)
  circle A6 centre (-25.146, 17.526) radius 1.27
  circle A7 centre (-25.146, -17.526) radius 1.27
  line L56 (55.1434, -34.0614) -> (52.6034, -34.0614)
  line L57 (52.6034, -34.0614) -> (52.6034, -36.6014)
  line L58 (52.6034, -36.6014) -> (55.1434, -36.6014)
  line L59 (55.1434, -36.6014) -> (55.1434, -34.0614)
  line L60 (52.6034, -36.6014) -> (31.7754, -36.6014)
  line L61 (31.7754, -36.6014) -> (31.7754, -112.8014)
  line L62 (31.7754, -112.8014) -> (52.6034, -112.8014)
  line L63 (52.6034, -112.8014) -> (52.6034, -36.6014)
  line L64 (-55.1434, -34.0614) -> (-52.6034, -34.0614)
  line L65 (-52.6034, -34.0614) -> (-52.6034, -36.6014)
  line L66 (-52.6034, -36.6014) -> (-55.1434, -36.6014)
  line L67 (-55.1434, -36.6014) -> (-55.1434, -34.0614)
  line L68 (-52.6034, -36.6014) -> (-31.7754, -36.6014)
  line L69 (-31.7754, -36.6014) -> (-31.7754, -112.8014)
  line L70 (-31.7754, -112.8014) -> (-52.6034, -112.8014)
  line L71 (-52.6034, -112.8014) -> (-52.6034, -36.6014)
  dimension "d157" = 2.54
  dimension "d158" = 2.54
  dimension "d159" = 20.828
  dimension "d160" = 76.2
  dimension "d161" = 2.54
  dimension "d162" = 2.54
  dimension "d163" = 20.828
  dimension "d164" = 76.2
  constraint horizontal L56
  constraint vertical L57
  constraint horizontal L58
  constraint vertical L59
  constraint coincident L4.end L5.start
  constraint horizontal L60
  constraint vertical L61
  constraint horizontal L62
  constraint vertical L63
  constraint horizontal L64
  constraint vertical L65
  constraint horizontal L66
  constraint vertical L67
  constraint coincident L37.end L38.start
  constraint horizontal L68
  constraint vertical L69
  constraint horizontal L70
  constraint vertical L71
  measures "d157" distance of L4.end L56.end
  measures "d158" distance of L4.end L58.end
  measures "d159" distance of L57.end L60.end
  measures "d160" distance of L57.end L62.end
  measures "d161" distance of L37.end L64.end
  measures "d162" distance of L37.end L66.end
  measures "d163" distance of L65.end L68.end
  measures "d164" distance of L65.end L70.end
extrude "Extrude35" cut sketch "Sketch38" against normal blind 1.27 contours L60 L61 L62 L63 | L68 L69 L70 L71 bodies 1
move_body "Move3" bodies 2 3 4 5 to x (1, 0, 0) y (0, 1, 0) z (0, 0, 1) at (25.4, 0, 0)
hidden bodies 2 3 4 5
equation "d3 = ( ( 0.84 * 2 ) * 1 in ) + 0.3 in"
equation "d4 = 1.72 in + 0.2 in"
equation "d30 = ( ( 1.92 / 2 ) * 1 in )"
equation "d34 = 0.305 in + 0.1 in"
equation "d46 = ( 1.92 / 2 ) * 1 in"
equation "d48 = 1.184 in + 0.2 in"
equation "d49 = 0.305 in + 0.1 in"
equation "d90 = 0.61 in + 0.1 in"
equation "d123 = ( 2.302 / 2 ) * 1 in"
equation "d124 = ( 2.302 / 2 ) * 1 in"
equation "d128 = 3.462 in + 0.1 in"
equation "d137 = ( 0.7 / 2 ) * 1 in"
equation "d138 = ( 0.7 / 2 ) * 1 in"
equation "d146 = 0.82 in + 0.1 in"
equation "d152 = 3.562 in / 2"
equation "d154 = 3 in + 0.2 in"
equation "d155 = 0.82 in + 0.1 in"
